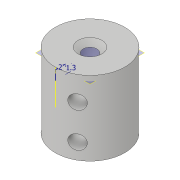
# Autodesk Inventor part: 00_Motorcoupling_5mm_M3
Saved by Autodesk Inventor 2019.4 (Build 234330000, 330)
## iProperties
Created: 2021-04-26
Part Number: 00_Motorcoupling_5mm_M3
Material: Generic
Document SubType Name: Modeling
Designer: diederichbenedict
Density: 1 g/cm^3
Appearance: Default
Mass: 1.15069 g
Surface Area: 11.4691 cm^2
Volume: 1.15069 cm^3
Author: diederichbenedict
Autodesk Inventor part; units mm, degrees
ref_plane "YZ Plane" through (0, 0, 0) normal (1, 0, 0) x (0, 1, 0)
ref_plane "XZ Plane" through (0, 0, 0) normal (0, 1, 0) x (-1, 0, 0)
ref_plane "XY Plane" through (0, 0, 0) normal (0, 0, 1) x (1, 0, 0)
sketch "Sketch1" plane through (0, 0, 0) normal (0, 1, 0) x (-1, 0, 0)
  circle A0 centre (0, 0) radius 7
  line L0 (0, -9.8) -> (0, 9.8) construction
  circle A1 centre (0, 0) radius 1.4
  dimension "d0" = 14
  dimension "d42" = 2.8
  constraints: 2 centre point, 1 coincident
  measures "d0" diameter of A0
  measures "d42" diameter of A1
extrude "Extrusion1" add sketch "Sketch1" along normal blind 7
sketch "Sketch2" plane through (0, 0, 0) normal (0, -1, 0) x (1, 0, 0)
  circle A0 centre (0, 0) radius 1.45 projected
  arc A1 (1.2894, -2.2) -> (-1.2894, -2.2) centre (0, 0) ccw
  line L0 (-1.2894, -2.2) -> (1.2894, -2.2)
  circle A2 centre (0, 0) radius 7 projected
  dimension "d4" = 5.1
  dimension "d5" = 2.2
  constraints: 2 end point, 2 point on circle, 1 centre point, 1 coincident, 1 horizontal
  measures "d4" diameter of A1
  measures "d5" distance from line of L0 point (0, 0)
extrude "Extrusion2" add sketch "Sketch2" along normal blind 8 contours A2
ref_plane "Work Plane1" through (0, 6, 0) normal (0, -1, 0) x (1, 0, 0)
sketch "Sketch5" plane through (0, 0, 0) normal (1, 0, 0) x (0, 1, 0)
  line L0 (0, 7) -> (7, 7) projected
  line L1 (4.6942, 7) -> (5.9942, 7)
  line L2 (5.9942, 7) -> (5.9942, 5)
  line L3 (5.9942, 5) -> (4.6942, 5)
  line L4 (4.6942, 5) -> (4.6942, 7)
  point P0 (0, 0)
  dimension "d17" = 1.3
  dimension "d18" = 2
  constraints: 8 end point, 2 parallel, 1 horizontal, 1 perpendicular, 1 point on line
  measures "d17" distance of L2.end L3.end
  measures "d18" distance of L1.end L2.end
sketch "Sketch6" plane through (0, 0, 0) normal (1, 0, 0) x (0, 1, 0)
  circle A0 centre (2.1729, 0) radius 1.45
  line L0 (-8, -7) -> (7, -7) projected
  point P0 (0, 0)
  dimension "d43" = 2.9
  dimension "d44" = 7
  constraints: 1 centre point
  measures "d43" diameter of A0
  measures "d44" distance from line of A0.centre L0
extrude "Extrusion5" cut sketch "Sketch6" against normal blind 10
pattern_circular "Circular Pattern3" count 3 over 360 about axis through (0, 0, 0) along (0, 1, 0) of "Extrusion5"
chamfer "Chamfer4" distance 1 angle 45 3 edges at (1.4, 7, 0) (0, -8, 2.55) (0, -8, -2.2)
pattern_linear "Rectangular Pattern2" count 2 spacing 7 along (0, -1, 0) of "Extrusion5", "Circular Pattern3"
body "Solid1"
